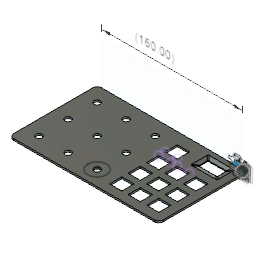
mymidicontroller (Autodesk Fusion 360 design; units mm, degrees)
part number: 2026-08-06-12-45-41-312
Autodesk Fusion 360 part; units mm, degrees
sketch "Sketch1" plane through (0, 0, 0) normal (0, 0, 1) x (1, 0, 0)
  line L0 (0, 0) -> (170, 0)
  line L1 (170, 0) -> (170, 100)
  line L2 (170, 100) -> (0, 100)
  line L3 (0, 100) -> (0, 0)
  dimension "d1" = 170
  dimension "d2" = 100
  constraint horizontal L0
  constraint vertical L1
  constraint horizontal L2
  constraint vertical L3
  constraint coincident L0.start L3.end
  measures "d1" distance of L0.start L0.end
  measures "d2" distance of L0.start L2.end
extrude "Extrude1" add sketch "Sketch1" along normal blind 2 makes body 1
sketch "Sketch2" plane through (0, 0, 2) normal (0, 0, 1) x (-1, 0, 0)
  line L0 (0, -100) -> (0, 0)
  line L1 (0, 0) -> (-170, 0)
  line L2 (-170, 0) -> (-170, -100)
  line L3 (-170, -100) -> (0, -100)
  circle A0 centre (-17, -83) radius 3.5
  circle A1 centre (-50, -83) radius 3.5
  circle A2 centre (-83, -83) radius 3.5
  circle A3 centre (-17, -50) radius 3.5
  circle A4 centre (-50, -50) radius 3.5
  circle A5 centre (-83, -50) radius 3.5
  circle A6 centre (-17, -17) radius 3.5
  circle A7 centre (-50, -17) radius 3.5
  circle A8 centre (-83, -17) radius 3.5
  line L4 (-146.2, -23.8) -> (-160, -23.8)
  line L5 (-160, -23.8) -> (-160, -10)
  line L6 (-160, -10) -> (-146.2, -10)
  line L7 (-146.2, -10) -> (-146.2, -23.8)
  dimension "d5" = 7
  dimension "d9" = -66
  dimension "d10" = 66
  dimension "d11" = 100
  dimension "d12" = 33
  dimension "d13" = 17
  dimension "d14" = 17
  dimension "d15" = 17
  dimension "d16" = 13.8
  dimension "d17" = 13.8
  dimension "d18" = 10
  dimension "d19" = 10
  constraint horizontal L4
  constraint vertical L5
  constraint horizontal L6
  constraint vertical L7
  measures "d5" diameter of A0
  measures "d11" distance of L1 L3
  measures "d12" distance of A0.centre A3.centre
  measures "d13" distance of L3 A0.centre
  measures "d14" distance of L1 A6.centre
  measures "d15" distance of L0 A0.centre
  measures "d16" distance of L4.start L4.end
  measures "d17" distance of L4.start L6.end
  measures "d18" distance of L1 L6
  measures "d19" distance of L2 L5
sketch "Sketch3" plane through (0, 0, 2) normal (0, 0, 1) x (-1, 0, 0)
hole "Hole1" at (17, 83, 2) at (50, 83, 2) at (83, 83, 2) at (83, 50, 2) at (83, 17, 2) at (50, 17, 2) at (17, 17, 2) at (17, 50, 2) at (50, 50, 2) direction (0, 0, -1) diameter 7 depth 2 tip angle 180 bodies 1
sketch "Sketch4" plane through (0, 0, 2) normal (0, 0, 1) x (-1, 0, 0)
  line L0 (0, -100) -> (0, 0)
  line L1 (0, 0) -> (-170, 0)
  line L2 (-170, 0) -> (-170, -100)
  line L3 (-170, -100) -> (0, -100)
  circle A0 centre (-50, -50) radius 3.5
  circle A1 centre (-17, -17) radius 3.5
  circle A2 centre (-83, -17) radius 3.5
  circle A3 centre (-83, -83) radius 3.5
  circle A4 centre (-17, -83) radius 3.5
  circle A5 centre (-50, -83) radius 3.5
  circle A6 centre (-83, -50) radius 3.5
  circle A7 centre (-50, -17) radius 3.5
  circle A8 centre (-17, -50) radius 3.5
  line L4 (-160, -10) -> (-146.2, -10)
  line L5 (-146.2, -10) -> (-146.2, -23.8)
  line L6 (-146.2, -23.8) -> (-160, -23.8)
  line L7 (-160, -23.8) -> (-160, -10)
  dimension "d23" = 13.8
  dimension "d24" = 13.8
  dimension "d25" = 10
  dimension "d26" = 10
  constraint horizontal L4
  constraint vertical L5
  constraint horizontal L6
  constraint vertical L7
  measures "d23" distance of L4.start L4.end
  measures "d24" distance of L4.start L6.end
  measures "d25" distance of L1 L4
  measures "d26" distance of L2 L7
sketch "Sketch5" plane through (0, 0, 2) normal (0, 0, 1) x (-1, 0, 0)
extrude "Extrude2" cut sketch "Sketch4" against normal blind 2 contours L4 L5 L6 L7 bodies 1
pattern_linear "R-Pattern1" count 3 spacing 21 along (-1, 0, 0) count 3 spacing 21 along (0, 1, 0) of "Extrude2"
sketch "Sketch6" plane through (0, 0, 2) normal (0, 0, 1) x (-1, 0, 0)
  line L0 (-146.2, -10) -> (-146.2, -23.8)
  line L1 (-146.2, -23.8) -> (-160, -23.8)
  line L2 (-160, -23.8) -> (-160, -10)
  line L3 (-160, -10) -> (-146.2, -10)
  line L4 (0, -100) -> (0, 0)
  line L5 (0, 0) -> (-170, 0)
  line L6 (-170, 0) -> (-170, -100)
  line L7 (-170, -100) -> (0, -100)
  circle A0 centre (-50, -50) radius 3.5
  circle A1 centre (-17, -17) radius 3.5
  circle A2 centre (-83, -17) radius 3.5
  circle A3 centre (-83, -83) radius 3.5
  circle A4 centre (-17, -83) radius 3.5
  circle A5 centre (-50, -83) radius 3.5
  circle A6 centre (-83, -50) radius 3.5
  circle A7 centre (-50, -17) radius 3.5
  circle A8 centre (-17, -50) radius 3.5
  line L8 (-125.2, -10) -> (-125.2, -23.8)
  line L9 (-125.2, -23.8) -> (-139, -23.8)
  line L10 (-139, -23.8) -> (-139, -10)
  line L11 (-139, -10) -> (-125.2, -10)
  line L12 (-104.2, -10) -> (-104.2, -23.8)
  line L13 (-104.2, -23.8) -> (-118, -23.8)
  line L14 (-118, -23.8) -> (-118, -10)
  line L15 (-118, -10) -> (-104.2, -10)
  line L16 (-146.2, -31) -> (-146.2, -44.8)
  line L17 (-146.2, -44.8) -> (-160, -44.8)
  line L18 (-160, -44.8) -> (-160, -31)
  line L19 (-160, -31) -> (-146.2, -31)
  line L20 (-125.2, -31) -> (-125.2, -44.8)
  line L21 (-125.2, -44.8) -> (-139, -44.8)
  line L22 (-139, -44.8) -> (-139, -31)
  line L23 (-139, -31) -> (-125.2, -31)
  line L24 (-104.2, -31) -> (-104.2, -44.8)
  line L25 (-104.2, -44.8) -> (-118, -44.8)
  line L26 (-118, -44.8) -> (-118, -31)
  line L27 (-118, -31) -> (-104.2, -31)
  line L28 (-146.2, -52) -> (-146.2, -65.8)
  line L29 (-146.2, -65.8) -> (-160, -65.8)
  line L30 (-160, -65.8) -> (-160, -52)
  line L31 (-160, -52) -> (-146.2, -52)
  line L32 (-125.2, -52) -> (-125.2, -65.8)
  line L33 (-125.2, -65.8) -> (-139, -65.8)
  line L34 (-139, -65.8) -> (-139, -52)
  line L35 (-139, -52) -> (-125.2, -52)
  line L36 (-104.2, -52) -> (-104.2, -65.8)
  line L37 (-104.2, -65.8) -> (-118, -65.8)
  line L38 (-118, -65.8) -> (-118, -52)
  line L39 (-118, -52) -> (-104.2, -52)
  circle A9 centre (-83, -17) radius 10.5
  dimension "d33" = 21
  constraint concentric A2 A9
  measures "d33" diameter of A9
  measures "d74" radius of L36.start
sketch "Sketch7" plane through (0, 0, 2) normal (0, 0, 1) x (-1, 0, 0)
  line L0 (-133, -96.2) -> (-160, -96.2)
  line L1 (-160, -96.2) -> (-160, -69.2)
  line L2 (-160, -69.2) -> (-133, -69.2)
  line L3 (-133, -69.2) -> (-133, -96.2)
  line L4 (-170, -100) -> (0, -100)
  line L5 (-160, -10) -> (-146.2, -10)
  line L6 (0, 0) -> (-170, 0)
  line L7 (-136, -90) -> (-157, -90)
  line L8 (-157, -90) -> (-157, -79.2)
  line L9 (-157, -79.2) -> (-136, -79.2)
  line L10 (-136, -79.2) -> (-136, -90)
  line L11 (-170, 0) -> (-170, -100)
  line L12 (-146.2, -65.8) -> (-160, -65.8)
  dimension "d36" = 27
  dimension "d37" = 27
  dimension "d38" = 3.8
  dimension "d39" = 10
  dimension "d40" = 3
  dimension "d42" = 10.8
  dimension "d43" = 21
  dimension "d53" = 10
  dimension "d55" = 10
  dimension "d67" = 6.2
  dimension "d68" = 10
  dimension "d69" = 3.4
  constraint horizontal L0
  constraint vertical L1
  constraint horizontal L2
  constraint vertical L3
  constraint horizontal L7
  constraint vertical L8
  constraint horizontal L9
  constraint vertical L10
  measures "d36" distance of L0.start L0.end
  measures "d37" distance of L0.start L2.end
  measures "d38" distance of L0 L4
  measures "d39" distance of L5 L6
  measures "d40" distance of L3 L10
  measures "d42" distance of L7.end L8.end
  measures "d43" distance of L8.end L9.end
  measures "d53" distance of L1 L11
  measures "d55" distance of L4 L7
  measures "d67" distance of L0 L7
  measures "d68" distance of L2 L9
  measures "d69" distance of L2 L12
extrude "Extrude3" cut sketch "Sketch7" against normal blind 2 contours L7 L8 L9 L10 bodies 1
chamfer "Chamfer1" distance 4.5 distance2 1 4 edges at (146.5, 90, 2) (136, 84.6, 2) (146.5, 79.2, 2) (157, 84.6, 2) measured on face at (108.8707, 79.8596, 2) measured on face at (108.8707, 79.8596, 2) measured on face at (108.8707, 79.8596, 2) measured on face at (108.8707, 79.8596, 2) on bodies 1
sketch "Sketch8" plane through (0, 0, 2) normal (0, 0, 1) x (-1, 0, 0)
  line L0 (-104.2, -86.8) -> (-118, -86.8)
  line L1 (-118, -86.8) -> (-118, -73)
  line L2 (-118, -73) -> (-104.2, -73)
  line L3 (-104.2, -73) -> (-104.2, -86.8)
  line L4 (-118, -52) -> (-104.2, -52)
  line L5 (-125.2, -52) -> (-125.2, -65.8)
  point P0 (-104.2, -10)
  point P1 (-125.2, -10)
  dimension "d48" = 21
  dimension "d49" = 21
  dimension "d50" = 21
  dimension "d51" = 13.8
  dimension "d52" = 13.8
  constraint horizontal L0
  constraint vertical L1
  constraint horizontal L2
  constraint vertical L3
  measures "d48" distance of P0 P1
  measures "d49" distance of L2 L4
  measures "d50" distance of L3 L5
  measures "d51" distance of L0.start L0.end
  measures "d52" distance of L0.end L1.end
extrude "Extrude4" cut sketch "Sketch8" against normal blind 2 bodies 1
sketch "Sketch9" plane through (0, 0, 2) normal (0, 0, 1) x (-1, 0, 0)
  line L0 (-125.2, -65.8) -> (-139, -65.8)
  line L1 (-118, -73) -> (-104.2, -73)
  line L2 (-104.2, -65.8) -> (-118, -65.8)
  dimension "d61" = 7.2
  measures "d61" distance of L1 L2
fillet "Fillet1" radius 5 4 edges at (170, 0, 1) (170, 100, 1) (0, 0, 1) (0, 100, 1) on bodies 1
fillet "Fillet2" radius 5 4 edges at (133.75, 92.25, 1.5) (133.75, 76.95, 1.5) (159.25, 92.25, 1.5) (159.25, 76.95, 1.5) on bodies 1
sketch "Sketch10" plane through (0, 0, 2) normal (0, 0, 1) x (-1, 0, 0)
  line L0 (-5, 0) -> (-165, 0)
  line L1 (-170, -5) -> (-170, -95)
  line L2 (-165, -100) -> (-5, -100)
  line L3 (0, -95) -> (0, -5)
  line L4 (-3, -102) -> (-167, -102)
  line L5 (-172, -97) -> (-172, -3)
  line L6 (-167, 2) -> (-3, 2)
  line L7 (2, -3) -> (2, -97)
  arc A0 (-5, -100) -> (0, -95) centre (-5, -95) ccw
  arc A1 (-170, -95) -> (-165, -100) centre (-165, -95) ccw
  arc A2 (-165, 0) -> (-170, -5) centre (-165, -5) ccw
  arc A3 (0, -5) -> (-5, 0) centre (-5, -5) ccw
  arc A4 (2, -3) -> (-3, 2) centre (-3, -3) ccw
  arc A5 (-3, -102) -> (2, -97) centre (-3, -97) ccw
  arc A6 (-172, -97) -> (-167, -102) centre (-167, -97) ccw
  arc A7 (-167, 2) -> (-172, -3) centre (-167, -3) ccw
  dimension "d70" = 2
  dimension "d71" = 2
  dimension "d72" = 2
  dimension "d73" = 2
  dimension "d74" = 5
  constraint horizontal L0
  constraint vertical L1
  constraint horizontal L2
  constraint vertical L3
  constraint horizontal L4
  constraint vertical L5
  constraint horizontal L6
  constraint vertical L7
  constraint tangent L2 A0
  constraint tangent L3 A0
  constraint tangent L1 A1
  constraint tangent L2 A1
  constraint equal A0 A1
  constraint tangent L0 A2
  constraint tangent L1 A2
  constraint equal A0 A2
  constraint tangent L0 A3
  constraint tangent L3 A3
  constraint equal A0 A3
  constraint tangent L6 A4
  constraint tangent L7 A4
  constraint equal A0 A4
  constraint tangent L4 A5
  constraint tangent L7 A5
  constraint equal A0 A5
  constraint tangent L4 A6
  constraint tangent L5 A6
  constraint equal A0 A6
  constraint tangent L5 A7
  constraint tangent L6 A7
  constraint equal A0 A7
  measures "d70" distance of L0 L6
  measures "d71" distance of L1 L5
  measures "d72" distance of L2 L4
  measures "d73" distance of L3 L7
  measures "d74" radius of A0
extrude "Extrude5" add sketch "Sketch10" along normal blind 50 separate body makes body 2
move_face "OffsetFaces1" offset 2 1 faces at (58.3333, -1.3333, 2) on bodies 2
sketch "Sketch11" plane through (0, 100, 0) normal (0, -1, 0) x (1, 0, 0)
  line L0 (5, 0) -> (165, 0)
  line L1 (165, 0) -> (165, 52)
  line L2 (165, 52) -> (5, 52)
  line L3 (5, 52) -> (5, 0)
  line L4 (165, 0.1269) -> (161.7551, 0.1269)
  line L5 (161.7551, 0.1269) -> (161.7551, 2.1269)
  line L6 (161.7551, 2.1269) -> (165, 2.1269)
  line L7 (165, 2.1269) -> (165, 0.1269)
  line L8 (161.7551, 2.1269) -> (156.7551, 2.1269)
  line L9 (156.7551, 2.1269) -> (156.7551, 4.1269)
  line L10 (156.7551, 4.1269) -> (161.7551, 4.1269)
  line L11 (161.7551, 4.1269) -> (161.7551, 2.1269)
  dimension "d78" = 2
  dimension "d79" = 5
  dimension "d80" = 2
  dimension "d81" = 160
  constraint horizontal L4
  constraint vertical L5
  constraint horizontal L6
  constraint vertical L7
  constraint coincident L1 L4.start
  constraint horizontal L8
  constraint vertical L9
  constraint horizontal L10
  constraint vertical L11
  measures "d78" distance of L4.start L6.end
  measures "d79" distance of L5.end L8.end
  measures "d80" distance of L5.end L10.end
  measures "d81" distance of L1.end L2.end
hidden bodies 2
